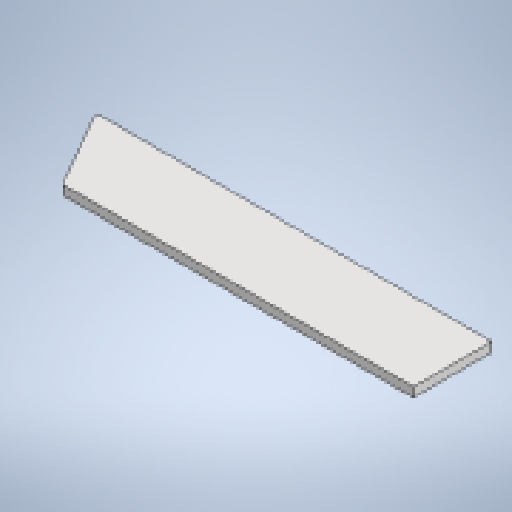
# Autodesk Inventor part: NVPH-410 feeder hose 3
Saved by Autodesk Inventor 2025 (Build 290162010, 162A)
## iProperties
Created: 2024-12-03
Part Number: NVPH-410 feeder hose 3
Material: Generic
Document SubType Name: Sheet Metal
Designer: admin
Density: 1 g/cm^3
Flat Pattern Width: 8.5 cm
Flat Pattern Length: 42.6 cm
Flat Pattern Area: 362.1 cm^2
Sheet Metal Rule: Default_mm
Sheet Metal Width: 85,000 mm
Sheet Metal Length: 426,000 mm
Sheet Metal Area: 36210,000 mm^2
Appearance: Default
Author: user
Autodesk Inventor part; units mm, degrees
ref_plane "YZ Plane" through (0, 0, 0) normal (1, 0, 0) x (0, 1, 0)
ref_plane "XZ Plane" through (0, 0, 0) normal (0, 1, 0) x (-1, 0, 0)
ref_plane "XY Plane" through (0, 0, 0) normal (0, 0, 1) x (1, 0, 0)
sketch "Sketch1" plane through (0, 0, 0) normal (0, 0, 1) x (1, 0, 0)
  line L0 (0, -42.5) -> (426, -42.5)
  line L1 (426, -42.5) -> (426, 42.5)
  line L2 (426, 42.5) -> (0, 42.5)
  line L3 (0, 42.5) -> (0, -42.5)
  line L4 (0, 37.5) -> (46.188, -42.5)
  point P0 (0, 0)
  point P1 (0, 50.9494)
  point P2 (0, 42.7975)
  point P3 (0, 0)
  dimension "d17" = 85
  dimension "d18" = 426
  dimension "d19" = 60
  dimension "d20" = 5
  measures "d17" distance of L0.end L1.end
  measures "d18" distance of L1.end L2.end
  measures "d19" angle of L2 L4
  measures "d20" distance of L2.end L4.start
extrude "Plate1" add sketch "Sketch1" along normal blind 10 contours L4 L3 L2 L1 L0
equation "\"d16\" = Thickness"
equation "\"BendReliefDepth\" = 0.5 * Thickness"
equation "\"Thickness\" = 10"
body "Solid2"
